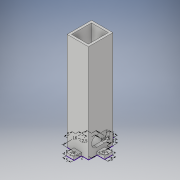
# Autodesk Inventor part: SoporteMotorx1
Saved by Autodesk Inventor 2019 (Build 230136000, 136)
## iProperties
Created: 2018-08-28
Part Number: SoporteMotorx1
Material: Genérico
Document SubType Name: Modeling
Designer: Cecilia Barrera Vill
Density: 1 g/cm^3
Appearance: Valor por defecto
Author: Cecilia Barrera Vill
Autodesk Inventor part; units mm, degrees
ref_plane "YZ Plane" through (0, 0, 0) normal (1, 0, 0) x (0, 1, 0)
ref_plane "XZ Plane" through (0, 0, 0) normal (0, 1, 0) x (-1, 0, 0)
ref_plane "XY Plane" through (0, 0, 0) normal (0, 0, 1) x (1, 0, 0)
sketch "Boceto1" plane through (0, 0, 0) normal (0, 1, 0) x (-1, 0, 0)
  line L0 (0, 0) -> (14, 0)
  line L1 (14, 0) -> (14, -16)
  line L2 (14, -16) -> (0, -16)
  line L3 (0, -16) -> (0, 0)
  line L4 (12, -2) -> (2, -2)
  line L5 (2, -2) -> (2, -14)
  line L6 (2, -14) -> (12, -14)
  line L7 (12, -14) -> (12, -2)
  line L8 (12, -2) -> (2, -14) construction
  line L9 (2, -2) -> (12, -14) construction
  line L10 (14, -8) -> (14, -10.5)
  line L11 (14, -10.5) -> (19, -10.5)
  line L12 (19, -10.5) -> (19, -5.5)
  line L13 (19, -5.5) -> (14, -5.5)
  circle A0 centre (16.5, -8) radius 1
  line L14 (7, -16) -> (4.5, -16)
  line L15 (4.5, -16) -> (4.5, -21)
  line L16 (4.5, -21) -> (9.5, -21)
  line L17 (9.5, -21) -> (9.5, -16)
  circle A1 centre (7, -18.5) radius 1
  line L18 (7, 0) -> (9.5, 0)
  line L19 (9.5, 0) -> (9.5, 5)
  line L20 (9.5, 5) -> (4.5, 5)
  line L21 (4.5, 5) -> (4.5, 0)
  circle A2 centre (7, 2.5) radius 1
  line L22 (0, -8) -> (0, -10.5)
  line L23 (0, -10.5) -> (-5, -10.5)
  line L24 (-5, -10.5) -> (-5, -5.5)
  line L25 (-5, -5.5) -> (0, -5.5)
  circle A3 centre (-2.5, -8) radius 1
  point P0 (7, -8)
  dimension "d0" = 14
  dimension "d1" = 16
  dimension "d2" = 10
  dimension "d3" = 12
  dimension "d4" = 2.5
  dimension "d5" = 5
  dimension "d6" = 5
  dimension "d7" = 2
  dimension "d8" = 2.5
  dimension "d9" = 5
  dimension "d10" = 5
  dimension "d11" = 2
  dimension "d12" = 2.5
  dimension "d13" = 5
  dimension "d14" = 5
  dimension "d15" = 2
  dimension "d16" = 2.5
  dimension "d17" = 5
  dimension "d18" = 5
  dimension "d19" = 2
  constraints: 52 end point, 14 perpendicular, 8 point on line, 6 midpoint, 4 centre point, 4 parallel, 2 horizontal
  measures "d0" distance of L1.end L2.end
  measures "d1" distance of L0.end L1.end
  measures "d2" distance of L6.end L5.end
  measures "d3" distance of L5.end L4.end
  measures "d4" distance of L10.start L10.end
  measures "d5" distance of L10.end L11.end
  measures "d6" distance of L11.end L12.end
  measures "d7" diameter of A0
  measures "d8" distance of L14.start L14.end
  measures "d9" distance of L14.end L15.end
  measures "d10" distance of L15.end L16.end
  measures "d11" diameter of A1
  measures "d12" distance of L18.start L18.end
  measures "d13" distance of L18.end L19.end
  measures "d14" distance of L19.end L20.end
  measures "d15" diameter of A2
  measures "d16" distance of L22.start L22.end
  measures "d17" distance of L22.end L23.end
  measures "d18" distance of L23.end L24.end
  measures "d19" diameter of A3
extrude "Extrusión1" add sketch "Boceto1" along normal blind 2
sketch "Boceto2" plane through (0, 2, 0) normal (0, 1, 0) x (1, 0, 0)
  line L0 (-9.5, 16) -> (-14, 16) projected
  line L1 (-14, 16) -> (0, 16)
  line L2 (0, 16) -> (0, 0)
  line L3 (-14, 0) -> (-9.5, 0) projected
  line L4 (0, 0) -> (-14, 0)
  line L5 (-14, 16) -> (-14, 10.5) projected
  line L6 (-14, 0) -> (-14, 16)
  line L7 (-2, 14) -> (-12, 14) projected
  line L8 (-12, 14) -> (-12, 1.9304)
  line L9 (-12, 1.9304) -> (-2, 1.9304)
  line L10 (-2, 14) -> (-2, 2) projected
  line L11 (-2, 1.9304) -> (-2, 14)
  line L12 (-2, 14) -> (-12, 14)
  constraints: 16 end point, 4 perpendicular, 2 collinear, 1 horizontal, 1 vertical
extrude "Extrusión2" add sketch "Boceto2" along normal blind 62
sketch "Boceto3" plane through (0, 0, -10.5) normal (1, 0, 0) x (0, 0, -1)
  line L0 (-5, 7.8078) -> (0, 7.8078) construction
  line L1 (-5, 4.3078) -> (0, 4.3078)
  line L2 (0, 11.3078) -> (-5, 11.3078)
  arc A0 (-5, 11.3078) -> (-5, 4.3078) centre (-5, 7.8078) ccw
  arc A1 (0, 4.3078) -> (0, 11.3078) centre (0, 7.8078) ccw
  line L3 (3.5, 0) -> (3.5, 64) projected
  point P0 (-10.5, 0)
  point P1 (-2.5, 7.8078)
  constraints: 8 end point, 5 tangent, 4 point on circle, 2 centre point, 1 horizontal, 1 midpoint, 1 parallel
extrude "Extrusión3" cut sketch "Boceto3" against normal blind 2
extrude "Extrusión4" add sketch "Boceto1" along normal blind 2 contours L7 L6 L5 L4
sketch "Boceto4" plane through (0, 64, 0) normal (0, 1, 0) x (1, 0, 0)
  line L0 (-12, 14) -> (-2, 14) projected
  line L1 (-12, 14) -> (-2, 14)
  line L2 (-2, 2) -> (-2, 5.5) projected
  line L3 (-2, 14) -> (-2, 2)
  line L4 (-2, 1.9304) -> (-12, 1.9304) projected
  line L5 (-2, 2) -> (-12, 1.9304)
  line L6 (-12, 1.9304) -> (-12, 14)
  line L7 (-12.5, 14.4652) -> (-1.5, 14.4652)
  line L8 (-1.5, 14.4652) -> (-1.5, 1.4652)
  line L9 (-1.5, 1.4652) -> (-12.5, 1.4652)
  line L10 (-12.5, 1.4652) -> (-12.5, 14.4652)
  line L11 (-12.5, 14.4652) -> (-1.5, 1.4652) construction
  line L12 (-1.5, 14.4652) -> (-12.5, 1.4652) construction
  point P0 (0, 0)
  point P1 (-7, 7.9652)
  dimension "d28" = 11
  dimension "d29" = 13
  constraints: 20 end point, 2 horizontal, 2 midpoint, 2 parallel, 2 perpendicular
  measures "d28" distance of L8.end L9.end
  measures "d29" distance of L7.end L8.end
extrude "Extrusión5" cut sketch "Boceto4" against normal blind 28
